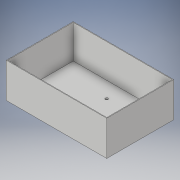
# Autodesk Inventor part: 546-1444-8-6x4-Enclosure
Saved by Autodesk Inventor 2018 (Build 220112000, 112)
## iProperties
Created: 2018-04-28
Part Number: 546-1444-8-6x4-Enclosure
Material: Generic
Document SubType Name: Modeling
Designer: bbramman
Density: 1 g/cm^3
Appearance: Default
Author: bbramman
Autodesk Inventor part; units mm, degrees
ref_plane "YZ Plane" through (0, 0, 0) normal (1, 0, 0) x (0, 1, 0)
ref_plane "XZ Plane" through (0, 0, 0) normal (0, 1, 0) x (-1, 0, 0)
ref_plane "XY Plane" through (0, 0, 0) normal (0, 0, 1) x (1, 0, 0)
sketch "Sketch1" plane through (0, 0, 0) normal (0, 1, 0) x (-1, 0, 0)
  line L0 (-76.2, 50.8) -> (76.2, 50.8)
  line L1 (76.2, 50.8) -> (76.2, -50.8)
  line L2 (76.2, -50.8) -> (-76.2, -50.8)
  line L3 (-76.2, -50.8) -> (-76.2, 50.8)
  line L4 (-76.2, 50.8) -> (76.2, -50.8) construction
  line L5 (76.2, 50.8) -> (-76.2, -50.8) construction
  point P0 (0, 0)
  dimension "d0" = 152.4
  dimension "d1" = 101.6
  constraints: 12 end point, 2 midpoint, 2 parallel, 1 horizontal, 1 perpendicular
  measures "d0" distance of L1.end L2.end
  measures "d1" distance of L0.end L1.end
extrude "Extrusion1" add sketch "Sketch1" along normal blind 2.032
sketch "Sketch2" plane through (0, 2.032, 0) normal (0, 1, 0) x (1, 0, 0)
  line L0 (-76.2, -50.8) -> (76.2, -50.8) projected
  line L1 (76.2, -50.8) -> (76.2, 50.8) projected
  line L2 (-76.2, -50.8) -> (76.2, -50.8)
  line L3 (76.2, -50.8) -> (76.2, 50.8)
  line L4 (76.2, 50.8) -> (-76.2, 50.8)
  line L5 (-76.2, 50.8) -> (-76.2, -50.8)
  line L6 (75.184, -49.784) -> (-75.184, -49.784)
  line L7 (-75.184, -49.784) -> (-75.184, 49.784)
  line L8 (-75.184, 49.784) -> (75.184, 49.784)
  line L9 (75.184, 49.784) -> (75.184, -49.784)
  line L10 (75.184, -49.784) -> (-75.184, 49.784) construction
  line L11 (-75.184, -49.784) -> (75.184, 49.784) construction
  point P0 (0, 0)
  dimension "d4" = 150.368
  dimension "d5" = 99.568
  constraints: 20 end point, 4 parallel, 2 horizontal, 2 midpoint, 2 perpendicular
  measures "d4" distance of L7.end L8.end
  measures "d5" distance of L6.end L7.end
extrude "Extrusion2" add sketch "Sketch2" along normal blind 50.8
sketch "Sketch3" plane through (0, 2.032, 0) normal (0, 1, 0) x (1, 0, 0)
  circle A0 centre (0, -25.4) radius 2.0828
  circle A1 centre (0, 25.4) radius 2.0828
  point P0 (0, 0)
  dimension "d10" = 4.1656
  dimension "d11" = 4.1656
  constraints: 2 centre point
  measures "d10" diameter of A0
  measures "d11" diameter of A1
extrude "Extrusion3" cut sketch "Sketch3" against normal through all
body "Solid1"
